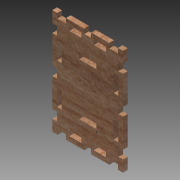
# Autodesk Inventor part: ceil_plate
Saved by Autodesk Inventor 2014 SP1 (Build 180222100, 222)
## iProperties
Created: 2013-12-24
Part Number: ceil_plate
Material: Wood (Birch)
Document SubType Name: Modeling
Designer: aoki
Density: 1 g/cm^3
Appearance: Birch - Natural Polished
Author: aoki
Autodesk Inventor part; units mm, degrees
ref_plane "YZ Plane" through (0, 0, 0) normal (1, 0, 0) x (0, 1, 0)
ref_plane "XZ Plane" through (0, 0, 0) normal (0, 1, 0) x (-1, 0, 0)
ref_plane "XY Plane" through (0, 0, 0) normal (0, 0, 1) x (1, 0, 0)
sketch "Block1" plane through (0, 0, 0) normal (0, 0, 1) x (1, 0, 0)
  line L0 (-50, 9) -> (-39, 9)
  line L1 (-39, 9) -> (-39, 4)
  line L2 (-39, 4) -> (-50, 4)
  line L3 (-50, 4) -> (-50, 9)
  line L4 (-39, -9) -> (-39, -4)
  line L5 (-50, -9) -> (-39, -9)
  line L6 (-50, -4) -> (-50, -9)
  line L7 (-39, -4) -> (-50, -4)
  line L8 (-39, 46) -> (-39, 41)
  line L9 (-50, 46) -> (-39, 46)
  line L10 (-50, 41) -> (-50, 46)
  line L11 (-39, 41) -> (-50, 41)
  line L12 (-39, -46) -> (-39, -41)
  line L13 (-50, -46) -> (-39, -46)
  line L14 (-50, -41) -> (-50, -46)
  line L15 (-39, -41) -> (-50, -41)
  point P0 (-44.5, 0)
  dimension "d59" = 11
  dimension "d60" = 5
  dimension "d62" = 11
  dimension "d63" = 5
  measures "d59" distance of L1.end L2.end
  measures "d60" distance of L0.end L1.end
  measures "d62" distance of L8.end L11.end
  measures "d63" distance of L9.end L8.end
sketch "Block2" plane through (0, 0, 0) normal (0, 0, 1) x (1, 0, 0)
  line L0 (-7.9, 59.1) -> (7.9, 59.1)
  line L1 (7.9, 59.1) -> (7.9, 50.1)
  line L2 (7.9, 50.1) -> (23.3, 50.1)
  line L3 (23.3, 50.1) -> (23.3, 59.1)
  line L4 (23.3, 59.1) -> (39.1, 59.1)
  line L5 (39.1, 59.1) -> (39.1, 50.1)
  line L6 (39.1, 50.1) -> (50.1, 50.1)
  line L7 (50.1, 50.1) -> (50.1, 41.9)
  line L8 (50.1, 41.9) -> (41.1, 41.9)
  line L9 (41.1, 41.9) -> (41.1, 36.1)
  line L10 (41.1, 36.1) -> (50.1, 36.1)
  line L11 (50.1, 36.1) -> (50.1, 12.9)
  line L12 (50.1, 12.9) -> (41.1, 12.9)
  line L13 (41.1, 12.9) -> (41.1, 7.1)
  line L14 (41.1, 7.1) -> (50.1, 7.1)
  line L15 (50.1, 7.1) -> (50.1, -7.1)
  line L16 (50.1, -7.1) -> (41.1, -7.1)
  line L17 (41.1, -7.1) -> (41.1, -12.9)
  line L18 (41.1, -12.9) -> (50.1, -12.9)
  line L19 (50.1, -12.9) -> (50.1, -36.1)
  line L20 (50.1, -36.1) -> (41.1, -36.1)
  line L21 (41.1, -36.1) -> (41.1, -41.9)
  line L22 (41.1, -41.9) -> (50.1, -41.9)
  line L23 (50.1, -41.9) -> (50.1, -50.1)
  line L24 (50.1, -50.1) -> (39.1, -50.1)
  line L25 (39.1, -50.1) -> (39.1, -59.1)
  line L26 (39.1, -59.1) -> (23.3, -59.1)
  line L27 (23.3, -59.1) -> (23.3, -50.1)
  line L28 (23.3, -50.1) -> (7.9, -50.1)
  line L29 (7.9, -50.1) -> (7.9, -59.1)
  line L30 (7.9, -59.1) -> (-7.9, -59.1)
  line L31 (-7.9, -59.1) -> (-7.9, -50.1)
  line L32 (-7.9, -50.1) -> (-23.3, -50.1)
  line L33 (-23.3, -50.1) -> (-23.3, -59.1)
  line L34 (-23.3, -59.1) -> (-39.1, -59.1)
  line L35 (-39.1, -59.1) -> (-39.1, -50.1)
  line L36 (-39.1, -50.1) -> (-50.1, -50.1)
  line L37 (-50.1, -50.1) -> (-50.1, -41.9)
  line L38 (-50.1, -41.9) -> (-41.1, -41.9)
  line L39 (-41.1, -41.9) -> (-41.1, -36.1)
  line L40 (-41.1, -36.1) -> (-50.1, -36.1)
  line L41 (-50.1, -36.1) -> (-50.1, -12.9)
  line L42 (-50.1, -12.9) -> (-41.1, -12.9)
  line L43 (-41.1, -12.9) -> (-41.1, -7.1)
  line L44 (-41.1, -7.1) -> (-50.1, -7.1)
  line L45 (-50.1, -7.1) -> (-50.1, 7.1)
  line L46 (-50.1, 7.1) -> (-41.1, 7.1)
  line L47 (-41.1, 7.1) -> (-41.1, 12.9)
  line L48 (-41.1, 12.9) -> (-50.1, 12.9)
  line L49 (-50.1, 12.9) -> (-50.1, 36.1)
  line L50 (-50.1, 36.1) -> (-41.1, 36.1)
  line L51 (-41.1, 36.1) -> (-41.1, 41.9)
  line L52 (-41.1, 41.9) -> (-50.1, 41.9)
  line L53 (-50.1, 41.9) -> (-50.1, 50.1)
  line L54 (-50.1, 50.1) -> (-39.1, 50.1)
  line L55 (-39.1, 50.1) -> (-39.1, 59.1)
  line L56 (-39.1, 59.1) -> (-23.3, 59.1)
  line L57 (-23.3, 59.1) -> (-23.3, 50.1)
  line L58 (-23.3, 50.1) -> (-7.9, 50.1)
  line L59 (-7.9, 50.1) -> (-7.9, 59.1)
  line L60 (-29.9, 33.4333) -> (-39.1, 33.4333)
  line L61 (-39.1, 33.4333) -> (-39.1, 13.2333)
  line L62 (-39.1, 13.2333) -> (-29.9, 13.2333)
  line L63 (-29.9, 13.2333) -> (-29.9, 33.4333)
  line L64 (-29.9, -13.2333) -> (-39.1, -13.2333)
  line L65 (-39.1, -13.2333) -> (-39.1, -33.4333)
  line L66 (-39.1, -33.4333) -> (-29.9, -33.4333)
  line L67 (-29.9, -33.4333) -> (-29.9, -13.2333)
  line L68 (39.1, 33.4333) -> (39.1, 13.2333)
  line L69 (39.1, 13.2333) -> (29.9, 13.2333)
  line L70 (29.9, 13.2333) -> (29.9, 33.4333)
  line L71 (29.9, 33.4333) -> (39.1, 33.4333)
  line L72 (39.1, -13.2333) -> (29.9, -13.2333)
  line L73 (29.9, -13.2333) -> (29.9, -33.4333)
  line L74 (29.9, -33.4333) -> (39.1, -33.4333)
  line L75 (39.1, -33.4333) -> (39.1, -13.2333)
  point P0 (0, 0)
sketch "Block3" plane through (0, 0, 0) normal (0, 0, 1) x (1, 0, 0)
  line L0 (23.2, 59.2) -> (39.2, 59.2)
  line L1 (39.2, 59.2) -> (39.2, 50.2)
  line L2 (39.2, 50.2) -> (50.2, 50.2)
  line L3 (50.2, 50.2) -> (50.2, 41.8)
  line L4 (50.2, 41.8) -> (41.2, 41.8)
  line L5 (41.2, 41.8) -> (41.2, 36.2)
  line L6 (41.2, 36.2) -> (50.2, 36.2)
  line L7 (50.2, 36.2) -> (50.2, 12.8)
  line L8 (50.2, 12.8) -> (41.2, 12.8)
  line L9 (41.2, 12.8) -> (41.2, 7.2)
  line L10 (41.2, 7.2) -> (50.2, 7.2)
  line L11 (50.2, 7.2) -> (50.2, -7.2)
  line L12 (50.2, -7.2) -> (41.2, -7.2)
  line L13 (41.2, -7.2) -> (41.2, -12.8)
  line L14 (41.2, -12.8) -> (50.2, -12.8)
  line L15 (50.2, -12.8) -> (50.2, -36.2)
  line L16 (50.2, -36.2) -> (41.2, -36.2)
  line L17 (41.2, -36.2) -> (41.2, -41.8)
  line L18 (41.2, -41.8) -> (50.2, -41.8)
  line L19 (50.2, -41.8) -> (50.2, -50.2)
  line L20 (50.2, -50.2) -> (39.2, -50.2)
  line L21 (39.2, -50.2) -> (39.2, -59.2)
  line L22 (39.2, -59.2) -> (23.2, -59.2)
  line L23 (23.2, -59.2) -> (23.2, -50.2)
  line L24 (23.2, -50.2) -> (8, -50.2)
  line L25 (8, -50.2) -> (8, -59.2)
  line L26 (8, -59.2) -> (-8, -59.2)
  line L27 (-8, -59.2) -> (-8, -50.2)
  line L28 (-8, -50.2) -> (-23.2, -50.2)
  line L29 (-23.2, -50.2) -> (-23.2, -59.2)
  line L30 (-23.2, -59.2) -> (-39.2, -59.2)
  line L31 (-39.2, -59.2) -> (-39.2, -50.2)
  line L32 (-39.2, -50.2) -> (-50.2, -50.2)
  line L33 (-50.2, -50.2) -> (-50.2, -41.8)
  line L34 (-50.2, -41.8) -> (-41.2, -41.8)
  line L35 (-41.2, -41.8) -> (-41.2, -36.2)
  line L36 (-41.2, -36.2) -> (-50.2, -36.2)
  line L37 (-50.2, -36.2) -> (-50.2, -12.8)
  line L38 (-50.2, -12.8) -> (-41.2, -12.8)
  line L39 (-41.2, -12.8) -> (-41.2, -7.2)
  line L40 (-41.2, -7.2) -> (-50.2, -7.2)
  line L41 (-50.2, -7.2) -> (-50.2, 7.2)
  line L42 (-50.2, 7.2) -> (-41.2, 7.2)
  line L43 (-41.2, 7.2) -> (-41.2, 12.8)
  line L44 (-41.2, 12.8) -> (-50.2, 12.8)
  line L45 (-50.2, 12.8) -> (-50.2, 36.2)
  line L46 (-50.2, 36.2) -> (-41.2, 36.2)
  line L47 (-41.2, 36.2) -> (-41.2, 41.8)
  line L48 (-41.2, 41.8) -> (-50.2, 41.8)
  line L49 (-50.2, 41.8) -> (-50.2, 50.2)
  line L50 (-50.2, 50.2) -> (-39.2, 50.2)
  line L51 (-39.2, 50.2) -> (-39.2, 59.2)
  line L52 (-39.2, 59.2) -> (-23.2, 59.2)
  line L53 (-23.2, 59.2) -> (-23.2, 50.2)
  line L54 (-23.2, 50.2) -> (-8, 50.2)
  line L55 (-8, 50.2) -> (-8, 59.2)
  line L56 (-8, 59.2) -> (8, 59.2)
  line L57 (8, 59.2) -> (8, 50.2)
  line L58 (8, 50.2) -> (23.2, 50.2)
  line L59 (23.2, 50.2) -> (23.2, 59.2)
  line L60 (-29.8, 33.5333) -> (-39.2, 33.5333)
  line L61 (-39.2, 33.5333) -> (-39.2, 13.1333)
  line L62 (-39.2, 13.1333) -> (-29.8, 13.1333)
  line L63 (-29.8, 13.1333) -> (-29.8, 33.5333)
  line L64 (-29.8, -13.1333) -> (-39.2, -13.1333)
  line L65 (-39.2, -13.1333) -> (-39.2, -33.5333)
  line L66 (-39.2, -33.5333) -> (-29.8, -33.5333)
  line L67 (-29.8, -33.5333) -> (-29.8, -13.1333)
  line L68 (39.2, 33.5333) -> (39.2, 13.1333)
  line L69 (39.2, 13.1333) -> (29.8, 13.1333)
  line L70 (29.8, 13.1333) -> (29.8, 33.5333)
  line L71 (29.8, 33.5333) -> (39.2, 33.5333)
  line L72 (39.2, -13.1333) -> (29.8, -13.1333)
  line L73 (29.8, -13.1333) -> (29.8, -33.5333)
  line L74 (29.8, -33.5333) -> (39.2, -33.5333)
  line L75 (39.2, -33.5333) -> (39.2, -13.1333)
  point P0 (0, 0)
sketch "Block4" plane through (0, 0, 0) normal (0, 0, 1) x (1, 0, 0)
  line L0 (23.3, 59.1) -> (39.1, 59.1)
  line L1 (39.1, 59.1) -> (39.1, 50.1)
  line L2 (39.1, 50.1) -> (50.1, 50.1)
  line L3 (50.1, 50.1) -> (50.1, 41.9)
  line L4 (50.1, 41.9) -> (41.1, 41.9)
  line L5 (41.1, 41.9) -> (41.1, 36.1)
  line L6 (41.1, 36.1) -> (50.1, 36.1)
  line L7 (50.1, 36.1) -> (50.1, 12.9)
  line L8 (50.1, 12.9) -> (41.1, 12.9)
  line L9 (41.1, 12.9) -> (41.1, 7.1)
  line L10 (41.1, 7.1) -> (50.1, 7.1)
  line L11 (50.1, 7.1) -> (50.1, -7.1)
  line L12 (50.1, -7.1) -> (41.1, -7.1)
  line L13 (41.1, -7.1) -> (41.1, -12.9)
  line L14 (41.1, -12.9) -> (50.1, -12.9)
  line L15 (50.1, -12.9) -> (50.1, -36.1)
  line L16 (50.1, -36.1) -> (41.1, -36.1)
  line L17 (41.1, -36.1) -> (41.1, -41.9)
  line L18 (41.1, -41.9) -> (50.1, -41.9)
  line L19 (50.1, -41.9) -> (50.1, -50.1)
  line L20 (50.1, -50.1) -> (39.1, -50.1)
  line L21 (39.1, -50.1) -> (39.1, -59.1)
  line L22 (39.1, -59.1) -> (23.3, -59.1)
  line L23 (23.3, -59.1) -> (23.3, -50.1)
  line L24 (23.3, -50.1) -> (7.9, -50.1)
  line L25 (7.9, -50.1) -> (7.9, -59.1)
  line L26 (7.9, -59.1) -> (-7.9, -59.1)
  line L27 (-7.9, -59.1) -> (-7.9, -50.1)
  line L28 (-7.9, -50.1) -> (-23.3, -50.1)
  line L29 (-23.3, -50.1) -> (-23.3, -59.1)
  line L30 (-23.3, -59.1) -> (-39.1, -59.1)
  line L31 (-39.1, -59.1) -> (-39.1, -50.1)
  line L32 (-39.1, -50.1) -> (-50.1, -50.1)
  line L33 (-50.1, -50.1) -> (-50.1, -41.9)
  line L34 (-50.1, -41.9) -> (-41.1, -41.9)
  line L35 (-41.1, -41.9) -> (-41.1, -36.1)
  line L36 (-41.1, -36.1) -> (-50.1, -36.1)
  line L37 (-50.1, -36.1) -> (-50.1, -12.9)
  line L38 (-50.1, -12.9) -> (-41.1, -12.9)
  line L39 (-41.1, -12.9) -> (-41.1, -7.1)
  line L40 (-41.1, -7.1) -> (-50.1, -7.1)
  line L41 (-50.1, -7.1) -> (-50.1, 7.1)
  line L42 (-50.1, 7.1) -> (-41.1, 7.1)
  line L43 (-41.1, 7.1) -> (-41.1, 12.9)
  line L44 (-41.1, 12.9) -> (-50.1, 12.9)
  line L45 (-50.1, 12.9) -> (-50.1, 36.1)
  line L46 (-50.1, 36.1) -> (-41.1, 36.1)
  line L47 (-41.1, 36.1) -> (-41.1, 41.9)
  line L48 (-41.1, 41.9) -> (-50.1, 41.9)
  line L49 (-50.1, 41.9) -> (-50.1, 50.1)
  line L50 (-50.1, 50.1) -> (-39.1, 50.1)
  line L51 (-39.1, 50.1) -> (-39.1, 59.1)
  line L52 (-39.1, 59.1) -> (-23.3, 59.1)
  line L53 (-23.3, 59.1) -> (-23.3, 50.1)
  line L54 (-23.3, 50.1) -> (-7.9, 50.1)
  line L55 (-7.9, 50.1) -> (-7.9, 59.1)
  line L56 (-7.9, 59.1) -> (7.9, 59.1)
  line L57 (7.9, 59.1) -> (7.9, 50.1)
  line L58 (7.9, 50.1) -> (23.3, 50.1)
  line L59 (23.3, 50.1) -> (23.3, 59.1)
  line L60 (-29.9, 33.4333) -> (-39.1, 33.4333)
  line L61 (-39.1, 33.4333) -> (-39.1, 13.2333)
  line L62 (-39.1, 13.2333) -> (-29.9, 13.2333)
  line L63 (-29.9, 13.2333) -> (-29.9, 33.4333)
  line L64 (-29.9, -13.2333) -> (-39.1, -13.2333)
  line L65 (-39.1, -13.2333) -> (-39.1, -33.4333)
  line L66 (-39.1, -33.4333) -> (-29.9, -33.4333)
  line L67 (-29.9, -33.4333) -> (-29.9, -13.2333)
  line L68 (39.1, 33.4333) -> (39.1, 13.2333)
  line L69 (39.1, 13.2333) -> (29.9, 13.2333)
  line L70 (29.9, 13.2333) -> (29.9, 33.4333)
  line L71 (29.9, 33.4333) -> (39.1, 33.4333)
  line L72 (39.1, -13.2333) -> (29.9, -13.2333)
  line L73 (29.9, -13.2333) -> (29.9, -33.4333)
  line L74 (29.9, -33.4333) -> (39.1, -33.4333)
  line L75 (39.1, -33.4333) -> (39.1, -13.2333)
  point P0 (0, 0)
sketch "Block5" plane through (0, 0, 0) normal (0, 0, 1) x (1, 0, 0)
  line L0 (-7.18, 55.58) -> (7.18, 55.58)
  line L1 (7.18, 55.58) -> (7.18, 50.08)
  line L2 (7.18, 50.08) -> (21.22, 50.08)
  line L3 (21.22, 50.08) -> (21.22, 55.58)
  line L4 (21.22, 55.58) -> (35.58, 55.58)
  line L5 (35.58, 55.58) -> (35.58, 53.58)
  line L6 (35.58, 53.58) -> (46.58, 53.58)
  line L7 (46.58, 53.58) -> (46.58, 38.42)
  line L8 (46.58, 38.42) -> (41.08, 38.42)
  line L9 (41.08, 38.42) -> (41.08, 32.58)
  line L10 (41.08, 32.58) -> (46.58, 32.58)
  line L11 (46.58, 32.58) -> (46.58, 12.92)
  line L12 (46.58, 12.92) -> (41.08, 12.92)
  line L13 (41.08, 12.92) -> (41.08, 7.08)
  line L14 (41.08, 7.08) -> (46.58, 7.08)
  line L15 (46.58, 7.08) -> (46.58, -7.08)
  line L16 (46.58, -7.08) -> (41.08, -7.08)
  line L17 (41.08, -7.08) -> (41.08, -12.92)
  line L18 (41.08, -12.92) -> (46.58, -12.92)
  line L19 (46.58, -12.92) -> (46.58, -32.58)
  line L20 (46.58, -32.58) -> (41.08, -32.58)
  line L21 (41.08, -32.58) -> (41.08, -38.42)
  line L22 (41.08, -38.42) -> (46.58, -38.42)
  line L23 (46.58, -38.42) -> (46.58, -46.58)
  line L24 (46.58, -46.58) -> (35.58, -46.58)
  line L25 (35.58, -46.58) -> (35.58, -55.58)
  line L26 (35.58, -55.58) -> (21.22, -55.58)
  line L27 (21.22, -55.58) -> (21.22, -50.08)
  line L28 (21.22, -50.08) -> (7.18, -50.08)
  line L29 (7.18, -50.08) -> (7.18, -55.58)
  line L30 (7.18, -55.58) -> (-7.18, -55.58)
  line L31 (-7.18, -55.58) -> (-7.18, -50.08)
  line L32 (-7.18, -50.08) -> (-21.22, -50.08)
  line L33 (-21.22, -50.08) -> (-21.22, -55.58)
  line L34 (-21.22, -55.58) -> (-35.58, -55.58)
  line L35 (-35.58, -55.58) -> (-35.58, -46.58)
  line L36 (-35.58, -46.58) -> (-46.58, -46.58)
  line L37 (-46.58, -46.58) -> (-46.58, -38.42)
  line L38 (-46.58, -38.42) -> (-41.08, -38.42)
  line L39 (-41.08, -38.42) -> (-41.08, -32.58)
  line L40 (-41.08, -32.58) -> (-46.58, -32.58)
  line L41 (-46.58, -32.58) -> (-46.58, -12.92)
  line L42 (-46.58, -12.92) -> (-41.08, -12.92)
  line L43 (-41.08, -12.92) -> (-41.08, -7.08)
  line L44 (-41.08, -7.08) -> (-46.58, -7.08)
  line L45 (-46.58, -7.08) -> (-46.58, 7.08)
  line L46 (-46.58, 7.08) -> (-41.08, 7.08)
  line L47 (-41.08, 7.08) -> (-41.08, 12.92)
  line L48 (-41.08, 12.92) -> (-46.58, 12.92)
  line L49 (-46.58, 12.92) -> (-46.58, 32.58)
  line L50 (-46.58, 32.58) -> (-41.08, 32.58)
  line L51 (-41.08, 32.58) -> (-41.08, 38.42)
  line L52 (-41.08, 38.42) -> (-46.58, 38.42)
  line L53 (-46.58, 38.42) -> (-46.58, 53.58)
  line L54 (-46.58, 53.58) -> (-35.58, 53.58)
  line L55 (-35.58, 53.58) -> (-35.58, 55.58)
  line L56 (-35.58, 55.58) -> (-21.22, 55.58)
  line L57 (-21.22, 55.58) -> (-21.22, 50.08)
  line L58 (-21.22, 50.08) -> (-7.18, 50.08)
  line L59 (-7.18, 50.08) -> (-7.18, 55.58)
  line L60 (-29.92, 33.4133) -> (-35.58, 33.4133)
  line L61 (-35.58, 33.4133) -> (-35.58, 13.2533)
  line L62 (-35.58, 13.2533) -> (-29.92, 13.2533)
  line L63 (-29.92, 13.2533) -> (-29.92, 33.4133)
  line L64 (-29.92, -13.2533) -> (-35.58, -13.2533)
  line L65 (-35.58, -13.2533) -> (-35.58, -33.4133)
  line L66 (-35.58, -33.4133) -> (-29.92, -33.4133)
  line L67 (-29.92, -33.4133) -> (-29.92, -13.2533)
  line L68 (35.58, 33.4133) -> (35.58, 13.2533)
  line L69 (35.58, 13.2533) -> (29.92, 13.2533)
  line L70 (29.92, 13.2533) -> (29.92, 33.4133)
  line L71 (29.92, 33.4133) -> (35.58, 33.4133)
  line L72 (35.58, -13.2533) -> (29.92, -13.2533)
  line L73 (29.92, -13.2533) -> (29.92, -33.4133)
  line L74 (29.92, -33.4133) -> (35.58, -33.4133)
  line L75 (35.58, -33.4133) -> (35.58, -13.2533)
  point P0 (0, 0.3684)
sketch "Block6" plane through (0, 0, 0) normal (0, 0, 1) x (1, 0, 0)
  line L0 (-35.58, 55.58) -> (-21.22, 55.58)
  line L1 (-21.22, 55.58) -> (-21.22, 50.08)
  line L2 (-21.22, 50.08) -> (-7.18, 50.08)
  line L3 (-7.18, 50.08) -> (-7.18, 55.58)
  line L4 (-7.18, 55.58) -> (7.18, 55.58)
  line L5 (7.18, 55.58) -> (7.18, 50.08)
  line L6 (7.18, 50.08) -> (21.22, 50.08)
  line L7 (21.22, 50.08) -> (21.22, 55.58)
  line L8 (21.22, 55.58) -> (35.58, 55.58)
  line L9 (35.58, 55.58) -> (35.58, 53.58)
  line L10 (35.58, 53.58) -> (50.08, 53.58)
  line L11 (50.08, 53.58) -> (50.08, 37.92)
  line L12 (50.08, 37.92) -> (44.58, 37.92)
  line L13 (44.58, 37.92) -> (44.58, 32.08)
  line L14 (44.58, 32.08) -> (50.08, 32.08)
  line L15 (50.08, 32.08) -> (50.08, 12.92)
  line L16 (50.08, 12.92) -> (44.58, 12.92)
  line L17 (44.58, 12.92) -> (44.58, 7.08)
  line L18 (44.58, 7.08) -> (50.08, 7.08)
  line L19 (50.08, 7.08) -> (50.08, -7.08)
  line L20 (50.08, -7.08) -> (44.58, -7.08)
  line L21 (44.58, -7.08) -> (44.58, -12.92)
  line L22 (44.58, -12.92) -> (50.08, -12.92)
  line L23 (50.08, -12.92) -> (50.08, -32.08)
  line L24 (50.08, -32.08) -> (44.58, -32.08)
  line L25 (44.58, -32.08) -> (44.58, -37.92)
  line L26 (44.58, -37.92) -> (50.08, -37.92)
  line L27 (50.08, -37.92) -> (50.08, -46.58)
  line L28 (50.08, -46.58) -> (35.58, -46.58)
  line L29 (35.58, -46.58) -> (35.58, -55.58)
  line L30 (35.58, -55.58) -> (21.22, -55.58)
  line L31 (21.22, -55.58) -> (21.22, -50.08)
  line L32 (21.22, -50.08) -> (7.18, -50.08)
  line L33 (7.18, -50.08) -> (7.18, -55.58)
  line L34 (7.18, -55.58) -> (-7.18, -55.58)
  line L35 (-7.18, -55.58) -> (-7.18, -50.08)
  line L36 (-7.18, -50.08) -> (-21.22, -50.08)
  line L37 (-21.22, -50.08) -> (-21.22, -55.58)
  line L38 (-21.22, -55.58) -> (-35.58, -55.58)
  line L39 (-35.58, -55.58) -> (-35.58, -46.58)
  line L40 (-35.58, -46.58) -> (-50.08, -46.58)
  line L41 (-50.08, -46.58) -> (-50.08, -37.92)
  line L42 (-50.08, -37.92) -> (-44.58, -37.92)
  line L43 (-44.58, -37.92) -> (-44.58, -32.08)
  line L44 (-44.58, -32.08) -> (-50.08, -32.08)
  line L45 (-50.08, -32.08) -> (-50.08, -12.92)
  line L46 (-50.08, -12.92) -> (-44.58, -12.92)
  line L47 (-44.58, -12.92) -> (-44.58, -7.08)
  line L48 (-44.58, -7.08) -> (-50.08, -7.08)
  line L49 (-50.08, -7.08) -> (-50.08, 7.08)
  line L50 (-50.08, 7.08) -> (-44.58, 7.08)
  line L51 (-44.58, 7.08) -> (-44.58, 12.92)
  line L52 (-44.58, 12.92) -> (-50.08, 12.92)
  line L53 (-50.08, 12.92) -> (-50.08, 32.08)
  line L54 (-50.08, 32.08) -> (-44.58, 32.08)
  line L55 (-44.58, 32.08) -> (-44.58, 37.92)
  line L56 (-44.58, 37.92) -> (-50.08, 37.92)
  line L57 (-50.08, 37.92) -> (-50.08, 53.58)
  line L58 (-50.08, 53.58) -> (-35.58, 53.58)
  line L59 (-35.58, 53.58) -> (-35.58, 55.58)
  line L60 (-29.92, 33.4133) -> (-35.58, 33.4133)
  line L61 (-35.58, 33.4133) -> (-35.58, 13.2533)
  line L62 (-35.58, 13.2533) -> (-29.92, 13.2533)
  line L63 (-29.92, 13.2533) -> (-29.92, 33.4133)
  line L64 (-29.92, -13.2533) -> (-35.58, -13.2533)
  line L65 (-35.58, -13.2533) -> (-35.58, -33.4133)
  line L66 (-35.58, -33.4133) -> (-29.92, -33.4133)
  line L67 (-29.92, -33.4133) -> (-29.92, -13.2533)
  line L68 (35.58, 33.4133) -> (35.58, 13.2533)
  line L69 (35.58, 13.2533) -> (29.92, 13.2533)
  line L70 (29.92, 13.2533) -> (29.92, 33.4133)
  line L71 (29.92, 33.4133) -> (35.58, 33.4133)
  line L72 (35.58, -13.2533) -> (29.92, -13.2533)
  line L73 (29.92, -13.2533) -> (29.92, -33.4133)
  line L74 (29.92, -33.4133) -> (35.58, -33.4133)
  line L75 (35.58, -33.4133) -> (35.58, -13.2533)
  point P0 (0, 0.3684)
sketch "Sketch1" plane through (0, 0, 0) normal (0, 1, 0) x (-1, 0, 0)
  line L0 (35.5, -55.5) -> (-35.5, -55.5)
  line L1 (-35.5, -55.5) -> (-35.5, 55.5)
  line L2 (-35.5, 55.5) -> (35.5, 55.5)
  line L3 (35.5, 55.5) -> (35.5, -55.5)
  line L4 (35.5, -55.5) -> (-35.5, 55.5) construction
  line L5 (-35.5, -55.5) -> (35.5, 55.5) construction
  line L6 (0, -83.4858) -> (0, 82.8643) projected
  line L7 (94.3775, 0) -> (-215.5652, 0) projected
  point P0 (0, 0)
  point P1 (0, 0)
  point P2 (-20, 40)
  point P3 (20, 40)
  point P4 (-20, -40)
  point P5 (20, -40)
  dimension "d0" = 71
  dimension "d1" = 111
  dimension "d22" = 40
  dimension "d23" = 80
  constraints: 12 end point, 3 symmetric about line, 2 midpoint, 2 parallel, 1 coincident, 1 horizontal, 1 perpendicular
  measures "d0" distance of L1.end L2.end
  measures "d1" distance of L0.end L1.end
  measures "d22" distance of point (20, 40) point (-20, 40)
  measures "d23" distance of point (-20, -40) point (-20, 40)
extrude "Extrusion1" add sketch "Sketch1" along normal blind 5.5
sketch "Sketch6" plane through (0, 0, 0) normal (0, -1, 0) x (1, 0, 0)
  line L0 (35.5, 55.5) -> (-35.5, 55.5) projected
  line L1 (-35.5, 55.5) -> (-35.5, -55.5) projected
  line L2 (-35.5, 33.3333) -> (-30, 33.3333)
  line L3 (-30, 33.3333) -> (-30, 13.3333)
  line L4 (-30, 13.3333) -> (-35.5, 13.3333)
  line L5 (-35.5, 13.3333) -> (-35.5, 33.3333)
  line L6 (-21.3, 55.5) -> (-7.1, 55.5)
  line L7 (-7.1, 55.5) -> (-7.1, 50)
  line L8 (-7.1, 50) -> (-21.3, 50)
  line L9 (-21.3, 50) -> (-21.3, 55.5)
  line L10 (-94.3775, 0) -> (215.5652, 0) projected
  line L11 (0, -83.4858) -> (0, 82.8643) projected
  line L12 (-35.5, -33.3333) -> (-30, -33.3333)
  line L13 (-30, -33.3333) -> (-30, -13.3333)
  line L14 (-30, -13.3333) -> (-35.5, -13.3333)
  line L15 (-35.5, -13.3333) -> (-35.5, -33.3333)
  line L16 (21.3, 55.5) -> (7.1, 55.5)
  line L17 (7.1, 55.5) -> (7.1, 50)
  line L18 (7.1, 50) -> (21.3, 50)
  line L19 (21.3, 50) -> (21.3, 55.5)
  line L20 (35.5, 33.3333) -> (30, 33.3333)
  line L21 (30, 33.3333) -> (30, 13.3333)
  line L22 (30, 13.3333) -> (35.5, 13.3333)
  line L23 (35.5, 13.3333) -> (35.5, 33.3333)
  line L24 (30, -13.3333) -> (35.5, -13.3333)
  line L25 (35.5, -33.3333) -> (30, -33.3333)
  line L26 (35.5, -13.3333) -> (35.5, -33.3333)
  line L27 (30, -33.3333) -> (30, -13.3333)
  line L28 (-21.3, -55.5) -> (-7.1, -55.5)
  line L29 (-7.1, -55.5) -> (-7.1, -50)
  line L30 (-7.1, -50) -> (-21.3, -50)
  line L31 (-21.3, -50) -> (-21.3, -55.5)
  line L32 (7.1, -50) -> (21.3, -50)
  line L33 (21.3, -55.5) -> (7.1, -55.5)
  line L34 (21.3, -50) -> (21.3, -55.5)
  line L35 (7.1, -55.5) -> (7.1, -50)
  point P0 (0, 0)
  dimension "d38" = 5.5
  dimension "d39" = 5.5
  dimension "d40" = 22.1667
  dimension "d41" = 20
  dimension "d42" = 14.2
  dimension "d43" = 14.2
  constraints: 64 end point, 24 symmetric about line, 4 parallel, 2 horizontal, 2 perpendicular, 2 point on line
  measures "d38" distance of L2.start L2.end
  measures "d39" distance of L8.end L6.start
  measures "d40" distance between parallel lines of L0 L2
  measures "d41" distance of L2.end L3.end
  measures "d42" distance between parallel lines of L1 L9
  measures "d43" distance of L7.end L8.end
extrude "Extrusion2" cut sketch "Sketch6" against normal through all contours L19 L18 L17 L0 | L7 L8 L9 L0 | L2 L3 L4 L1 | L14 L13 L12 L1 | L23 L22 L21 L20 | L24 L26 L25 L27 | L31 L30 L29 L28 | L32 L34 L33 L35
sketch "Sketch26" plane through (0, 5.5, 0) normal (0, 1, 0) x (1, 0, 0)
  line L0 (-35.5, 55.5) -> (35.5, 55.5)
  line L1 (35.5, 55.5) -> (35.5, 61)
  line L2 (35.5, 61) -> (-35.5, 61)
  line L3 (-35.5, 61) -> (-35.5, 55.5)
  line L4 (0, 84.3) -> (0, -78.8) projected
  line L5 (-49.7, 0) -> (49.7, 0) projected
  line L6 (35.5, -55.5) -> (21.3, -55.5)
  line L7 (7.1, -55.5) -> (-7.1, -55.5)
  line L8 (-21.3, -55.5) -> (-35.5, -55.5)
  line L9 (-35.5, -55.5) -> (35.5, -55.5)
  line L10 (35.5, -55.5) -> (35.5, -61)
  line L11 (35.5, -61) -> (-35.5, -61)
  line L12 (-35.5, -61) -> (-35.5, -55.5)
  line L13 (-35.5, 61) -> (-41, 61)
  line L14 (-41, 61) -> (-41, -61)
  line L15 (-41, -61) -> (-35.5, -61)
  line L16 (-35.5, -61) -> (-35.5, 61)
  line L17 (35.5, 55.5) -> (35.5, 33.3333)
  line L18 (35.5, 13.3333) -> (35.5, -13.3333)
  line L19 (35.5, -33.3333) -> (35.5, -55.5)
  line L20 (35.5, 61) -> (35.5, 55.5)
  line L21 (35.5, -61) -> (35.5, -55.5)
  line L22 (35.5, 61) -> (41, 61)
  line L23 (41, 61) -> (41, -61)
  line L24 (41, -61) -> (35.5, -61)
  line L25 (35.5, -61) -> (35.5, 61)
  point P0 (35.5, 55.5)
  point P1 (0, 0)
  dimension "d126" = 5.5
  dimension "d127" = 5.5
  constraints: 48 end point, 8 symmetric about line, 4 parallel, 2 horizontal, 2 perpendicular
  measures "d126" distance of L0.end L1.end
  measures "d127" distance of L14.end L15.end
extrude "Extrusion13" add sketch "Sketch26" against normal blind 5.5 contours L3 L2 L4 L0 | L16 L5 L14 L13 L3 | L4 L2 L1 L0 | L16 L12 L15 L14 L5 | L1 L22 L23 L5 L18 L25 L17 | L8 L9 L7 L4 L11 L12 | L7 L9 L6 L10 L11 L4 | L5 L23 L24 L10 L19 L25 L18
sketch "Sketch27" plane through (0, 5.5, 0) normal (0, 1, 0) x (1, 0, 0)
  line L0 (-41, 61) -> (-41, -61) projected
  line L1 (-57.4, 0) -> (57.4, 0) projected
  line L2 (0, 85.4) -> (0, -85.4) projected
  line L3 (-41, 0) -> (-35.5, 0)
  line L4 (-35.5, 0) -> (-35.5, 5)
  line L5 (-35.5, 5) -> (-41, 5)
  line L6 (-41, 5) -> (-41, 0)
  line L7 (-35.5, 0) -> (-35.5, -5)
  line L8 (-35.5, -5) -> (-41, -5)
  line L9 (-41, -5) -> (-41, 0)
  line L10 (-41, 38) -> (-35.5, 38)
  line L11 (-35.5, 38) -> (-35.5, 48)
  line L12 (-35.5, 48) -> (-41, 48)
  line L13 (-41, 48) -> (-41, 38)
  line L14 (-41, -38) -> (-35.5, -38)
  line L15 (-35.5, -38) -> (-35.5, -48)
  line L16 (-35.5, -48) -> (-41, -48)
  line L17 (-41, -48) -> (-41, -38)
  line L18 (41, 0) -> (35.5, 0)
  line L19 (35.5, 0) -> (35.5, 5)
  line L20 (35.5, 5) -> (41, 5)
  line L21 (41, 5) -> (41, 0)
  line L22 (35.5, 0) -> (35.5, -5)
  line L23 (35.5, -5) -> (41, -5)
  line L24 (41, -5) -> (41, 0)
  line L25 (41, 38) -> (35.5, 38)
  line L26 (35.5, 38) -> (35.5, 48)
  line L27 (35.5, 48) -> (41, 48)
  line L28 (41, 48) -> (41, 38)
  line L29 (35.5, -38) -> (35.5, -48)
  line L30 (35.5, -48) -> (41, -48)
  line L31 (41, -48) -> (41, -38)
  line L32 (41, -38) -> (35.5, -38)
  line L33 (35.5, -33.3333) -> (35.5, -13.3333)
  line L34 (35.5, 13.3333) -> (35.5, 33.3333)
  point P0 (0, 0)
  dimension "d132" = 5
  dimension "d133" = 10
  dimension "d149" = 38
  constraints: 64 end point, 20 symmetric about line, 4 parallel, 2 horizontal, 2 perpendicular, 2 point on line, 1 midpoint
  measures "d132" distance of L4.end L3.end
  measures "d133" distance of L11.end L10.end
  measures "d149" distance between parallel lines of L1 L10
extrude "Extrusion15" cut sketch "Sketch27" against normal through all
sketch "Sketch28" plane through (0, 5.5, 0) normal (0, 1, 0) x (1, 0, 0)
  line L0 (41, 61) -> (-41, 61) projected
  line L1 (0, 61) -> (-4, 61)
  line L2 (-4, 61) -> (-4, 55.5)
  line L3 (-4, 55.5) -> (0, 55.5)
  line L4 (0, 55.5) -> (0, 61)
  line L5 (-57.4, 0) -> (57.4, 0) projected
  line L6 (0, 85.4) -> (0, -85.4) projected
  line L7 (0, 61) -> (4, 61)
  line L8 (4, 61) -> (4, 55.5)
  line L9 (4, 55.5) -> (0, 55.5)
  line L10 (-35, 61) -> (-25, 61)
  line L11 (-25, 61) -> (-25, 55.5)
  line L12 (-25, 55.5) -> (-35, 55.5)
  line L13 (-35, 55.5) -> (-35, 61)
  line L14 (35, 61) -> (25, 61)
  line L15 (25, 61) -> (25, 55.5)
  line L16 (25, 55.5) -> (35, 55.5)
  line L17 (35, 55.5) -> (35, 61)
  line L18 (0, -61) -> (-4, -61)
  line L19 (-4, -61) -> (-4, -55.5)
  line L20 (-4, -55.5) -> (0, -55.5)
  line L21 (0, -55.5) -> (0, -61)
  line L22 (4, -55.5) -> (0, -55.5)
  line L23 (4, -61) -> (4, -55.5)
  line L24 (0, -61) -> (4, -61)
  line L25 (-35, -61) -> (-25, -61)
  line L26 (-25, -61) -> (-25, -55.5)
  line L27 (-25, -55.5) -> (-35, -55.5)
  line L28 (-35, -55.5) -> (-35, -61)
  line L29 (25, -61) -> (25, -55.5)
  line L30 (35, -61) -> (25, -61)
  line L31 (35, -55.5) -> (35, -61)
  line L32 (25, -55.5) -> (35, -55.5)
  point P0 (-21.3, 55.5)
  point P1 (0, 0)
  point P2 (-21.3, -55.5)
  dimension "d139" = 4
  dimension "d140" = 5.5
  dimension "d141" = 10
  dimension "d142" = 5.5
  dimension "d148" = 25
  constraints: 60 end point, 21 symmetric about line, 4 parallel, 2 horizontal, 2 perpendicular, 1 midpoint, 1 point on line
  measures "d139" distance of L3.end L2.end
  measures "d140" distance of L2.end L1.end
  measures "d141" distance of L11.end L12.end
  measures "d142" distance of L10.end L11.end
  measures "d148" distance between parallel lines of L6 L11
extrude "Extrusion17" cut sketch "Sketch28" against normal through all
sketch "Sketch29" plane through (0, 0, 0) normal (0, -1, 0) x (1, 0, 0)
  line L0 (-57.4, 0) -> (57.4, 0) projected
  line L1 (0, -85.4) -> (0, 85.4) projected
  line L2 (-10, 27.25) -> (10, 27.25)
  line L3 (10, 27.25) -> (10, 32.75)
  line L4 (10, 32.75) -> (-10, 32.75)
  line L5 (-10, 32.75) -> (-10, 27.25)
  line L6 (-10, 27.25) -> (10, 32.75) construction
  line L7 (10, 27.25) -> (-10, 32.75) construction
  line L8 (-10, -27.25) -> (10, -27.25)
  line L9 (10, -27.25) -> (10, -32.75)
  line L10 (10, -32.75) -> (-10, -32.75)
  line L11 (-10, -32.75) -> (-10, -27.25)
  line L12 (-10, -27.25) -> (10, -32.75) construction
  line L13 (10, -27.25) -> (-10, -32.75) construction
  point P0 (0, 0)
  point P1 (0, 30)
  point P2 (0, -30)
  dimension "d150" = 20
  dimension "d151" = 5.5
  dimension "d152" = 60
  constraints: 24 end point, 5 symmetric about line, 4 midpoint, 2 parallel, 1 horizontal, 1 perpendicular, 1 point on line
  measures "d150" distance of L4.end L3.end
  measures "d151" distance of L3.end L2.end
  measures "d152" distance of point (0, -30) point (0, 30)
extrude "Extrusion18" cut sketch "Sketch29" against normal through all
equation "\"d2\" = Wt"
equation "\"d38\" = Wt"
equation "\"d39\" = Wt"
equation "\"d40\" = 0.166667 * d1 + 0.666667 * Wt"
equation "\"d41\" = -0.4 * Wt + 0.2 * d1"
equation "\"d42\" = 0.2 * d0"
equation "\"d43\" = 0.2 * d0"
equation "\"hogehoge\" = 9"
equation "\"Wt\" = 5.5"
body "Solid1"
